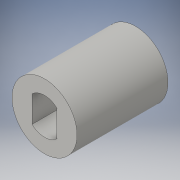
# Autodesk Inventor part: lazy susan motor test fit
Saved by Autodesk Inventor 2016 (Build 200138000, 138)
## iProperties
Created: 2018-09-10
Part Number: lazy susan motor test fit
Material: Generic
Document SubType Name: Modeling
Designer: student
Density: 1 g/cm^3
Appearance: Default
Author: student
Autodesk Inventor part; units mm, degrees
ref_plane "YZ Plane" through (0, 0, 0) normal (1, 0, 0) x (0, 1, 0)
ref_plane "XZ Plane" through (0, 0, 0) normal (0, 1, 0) x (-1, 0, 0)
ref_plane "XY Plane" through (0, 0, 0) normal (0, 0, 1) x (1, 0, 0)
sketch "Sketch1" plane through (0, 0, 0) normal (0, 0, 1) x (1, 0, 0)
  circle A0 centre (0, 0) radius 6.35
  line L0 (-2.4402, 2.5908) -> (2.4402, 2.5908)
  line L1 (2.4402, 2.5908) -> (2.4402, -2.5908)
  line L2 (2.4402, -2.5908) -> (-2.4402, -2.5908)
  line L3 (-2.4402, -2.5908) -> (-2.4402, 2.5908)
  line L4 (-2.4402, 2.5908) -> (2.4402, -2.5908) construction
  line L5 (2.4402, 2.5908) -> (-2.4402, -2.5908) construction
  arc A1 (2.4402, 2.5908) -> (-2.4402, 2.5908) centre (0, -0.0111) ccw
  arc A2 (-2.4402, -2.5908) -> (2.4402, -2.5908) centre (0, 0.0111) ccw
  dimension "d0" = 12.7
  dimension "d1" = 5.1816
  dimension "d2" = 4.8803
  dimension "d5" = 3.5671
  dimension "d6" = 3.5671
  constraints: 12 end point, 4 point on circle, 3 centre point, 2 midpoint, 2 parallel, 1 coincident, 1 horizontal, 1 perpendicular
  measures "d0" diameter of A0
  measures "d1" distance of L0.end L1.end
  measures "d2" distance between parallel lines of L1 L3
  measures "d5" radius of A1
  measures "d6" radius of A2
extrude "Extrusion1" add sketch "Sketch1" along normal blind 17.78
body "Solid1"
